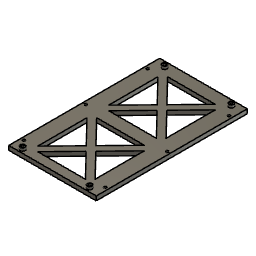
psu_base (Autodesk Fusion 360 design; units mm, degrees)
Autodesk Fusion 360 part; units mm, degrees
sketch "base" plane through (0, 0, 0) normal (0, 1, 0) x (1, 0, 0)
  line L0 (0, 0) -> (125, 0)
  line L1 (0, 0) -> (0, -245)
  line L2 (0, -245) -> (125, -245)
  line L3 (125, -245) -> (125, 0)
  line L4 (125, 0) -> (110, 0) construction
  line L5 (110, 0) -> (110, -15) construction
  line L6 (110, -15) -> (15, -15)
  line L7 (15, -15) -> (15, -230)
  line L8 (15, -230) -> (110, -230)
  line L9 (110, -230) -> (110, -15)
  line L10 (15, -122.5) -> (110, -122.5)
  line L11 (110, -122.5) -> (110, -132.5)
  line L12 (110, -132.5) -> (15, -132.5)
  line L13 (15, -132.5) -> (15, -122.5)
  line L14 (15, -122.5) -> (110, -122.5)
  line L15 (110, -122.5) -> (110, -112.5)
  line L16 (110, -112.5) -> (15, -112.5)
  line L17 (15, -112.5) -> (15, -122.5)
  line L18 (110, -112.5) -> (102, -112.5) construction
  line L19 (110, -112.5) -> (110, -104.5) construction
  line L20 (15, -15) -> (23, -15) construction
  line L21 (15, -15) -> (15, -23) construction
  line L22 (15, -23) -> (102, -112.5)
  line L23 (23, -15) -> (110, -104.5)
  line L24 (110, -15) -> (110, -23) construction
  line L25 (110, -15) -> (102, -15) construction
  line L26 (15, -112.5) -> (23, -112.5) construction
  line L27 (15, -112.5) -> (15, -104.5) construction
  line L28 (110, -23) -> (23, -112.5)
  line L29 (102, -15) -> (15, -104.5)
  line L30 (110, -132.5) -> (102, -132.5) construction
  line L31 (110, -132.5) -> (110, -140.5) construction
  line L32 (15, -132.5) -> (23, -132.5) construction
  line L33 (15, -132.5) -> (15, -140.5) construction
  line L34 (15, -230) -> (15, -222) construction
  line L35 (15, -230) -> (23, -230) construction
  line L36 (110, -230) -> (102, -230) construction
  line L37 (110, -230) -> (110, -222) construction
  line L38 (102, -132.5) -> (15, -222)
  line L39 (23, -230) -> (110, -140.5)
  line L40 (23, -132.5) -> (110, -222)
  line L41 (15, -140.5) -> (102, -230)
  line L42 (0, 0) -> (125, 0)
  line L43 (125, 0) -> (125, 5)
  line L44 (125, 5) -> (0, 5)
  line L45 (0, 5) -> (0, 0)
  dimension "d1" = 125
  dimension "d2" = 245
  dimension "d3" = 125
  dimension "d4" = 15
  dimension "d5" = 15
  dimension "d6" = 95
  dimension "d7" = 215
  dimension "d8" = 10
  dimension "d9" = 10
  dimension "d92" = 8
  dimension "d93" = 8
  dimension "d94" = 8
  dimension "d95" = 8
  dimension "d96" = 8
  dimension "d97" = 8
  dimension "d98" = 8
  dimension "d99" = 8
  dimension "d100" = 8
  dimension "d101" = 8
  dimension "d102" = 8
  dimension "d103" = 8
  dimension "d104" = 8
  dimension "d105" = 8
  dimension "d106" = 8
  dimension "d107" = 8
  dimension "d110" = 5
  constraint coincident L0.start L1.start
  constraint horizontal L0
  constraint perpendicular L0 L1
  constraint perpendicular L1 L2
  constraint perpendicular L3 L4
  constraint perpendicular L4 L5
  constraint horizontal L6
  constraint vertical L7
  constraint horizontal L8
  constraint vertical L9
  constraint horizontal L10
  constraint vertical L11
  constraint horizontal L12
  constraint vertical L13
  constraint midpoint L7 L10.start
  constraint horizontal L14
  constraint vertical L15
  constraint horizontal L16
  constraint vertical L17
  constraint perpendicular L9 L18
  constraint perpendicular L16 L19
  constraint perpendicular L7 L20
  constraint perpendicular L6 L21
  constraint perpendicular L6 L24
  constraint perpendicular L5 L25
  constraint perpendicular L7 L26
  constraint perpendicular L26 L27
  constraint perpendicular L11 L30
  constraint perpendicular L12 L31
  constraint perpendicular L13 L32
  constraint perpendicular L12 L33
  constraint perpendicular L8 L34
  constraint perpendicular L34 L35
  constraint perpendicular L9 L36
  constraint perpendicular L8 L37
  constraint horizontal L42
  constraint vertical L43
  constraint horizontal L44
  constraint vertical L45
  measures "d1" distance of L0.start L0.end
  measures "d2" distance of L0.start L1.end
  measures "d3" distance of L1.end L2.end
  measures "d4" distance of L0.end L4.end
  measures "d5" distance of L4.end L5.end
  measures "d6" distance of L5.end L6.end
  measures "d7" distance of L5.end L8.end
  measures "d8" distance of L10.start L12.end
  measures "d9" distance of L10.start L16.end
  measures "d92" distance of L15.end L18.end
  measures "d93" distance of L15.end L19.end
  measures "d94" distance of L6.end L20.end
  measures "d95" distance of L6.end L21.end
  measures "d96" distance of L5.end L24.end
  measures "d97" distance of L5.end L25.end
  measures "d98" distance of L16.end L26.end
  measures "d99" distance of L16.end L27.end
  measures "d100" distance of L11.end L30.end
  measures "d101" distance of L11.end L31.end
  measures "d102" distance of L12.end L32.end
  measures "d103" distance of L12.end L33.end
  measures "d104" distance of L7.end L34.end
  measures "d105" distance of L7.end L35.end
  measures "d106" distance of L8.end L36.end
  measures "d107" distance of L8.end L37.end
  measures "d110" distance of L0.start L44.end
sketch "bolt" plane through (0, 0, 0) normal (0, 1, 0) x (1, 0, 0)
  line L0 (0, 0) -> (125, 0) construction
  line L1 (0, 0) -> (7.4, 0) construction
  line L2 (7.4, 0) -> (7.4, -4.25) construction
  circle A0 centre (7.4, -4.25) radius 2.125
  line L3 (125, 0) -> (118, 0) construction
  line L4 (118, 0) -> (118, -4.25) construction
  circle A1 centre (118, -4.25) radius 2.125
  circle A2 centre (7.4, -4.25) radius 4
  circle A3 centre (118, -4.25) radius 4
  line L5 (0, -245) -> (7, -245) construction
  line L6 (7, -245) -> (7, -239) construction
  circle A4 centre (7, -239) radius 4
  circle A5 centre (7, -239) radius 2.125
  line L7 (125, -245) -> (118, -245) construction
  line L8 (118, -245) -> (118, -239) construction
  circle A6 centre (118, -239) radius 4
  circle A7 centre (118, -239) radius 2.125
  point P0 (0, -245)
  point P1 (125, -245)
  dimension "d10" = 7.4
  dimension "d11" = 4.25
  dimension "d12" = 4.25
  dimension "d13" = 7
  dimension "d14" = 4.25
  dimension "d15" = 4.25
  dimension "d16" = 8
  dimension "d17" = 8
  dimension "d18" = 7
  dimension "d19" = 6
  dimension "d20" = 8
  dimension "d21" = 4.25
  dimension "d22" = 7
  dimension "d23" = 6
  dimension "d24" = 8
  dimension "d25" = 4.25
  constraint coincident L0.start L1.start
  constraint coincident L0 L1.end
  constraint perpendicular L1 L2
  constraint coincident L2.end A0.centre
  constraint coincident L0.end L3.start
  constraint perpendicular L0 L4
  constraint coincident L4.end A1.centre
  constraint concentric A0 A2
  constraint concentric A1 A3
  constraint coincident P0 L5.start
  constraint perpendicular L5 L6
  constraint coincident L6.end A4.centre
  constraint concentric A4 A5
  constraint coincident P1 L7.start
  constraint perpendicular L7 L8
  constraint coincident L8.end A6.centre
  constraint concentric A6 A7
  measures "d10" distance of L0.start L1.end
  measures "d11" diameter of A0
  measures "d12" distance of L1.end L2.end
  measures "d13" distance of L0.end L3.end
  measures "d14" distance of L3.end L4.end
  measures "d15" diameter of A1
  measures "d16" diameter of A2
  measures "d17" diameter of A3
  measures "d18" distance of P0 L5.end
  measures "d19" distance of L5.end L6.end
  measures "d20" diameter of A4
  measures "d21" diameter of A5
  measures "d22" distance of P1 L7.end
  measures "d23" distance of L7.end L8.end
  measures "d24" diameter of A6
  measures "d25" diameter of A7
extrude "Extrude1" add sketch "base" along normal blind 7 contours L0 L42 L43 L44 L45 | L0 L1 L2 L3 L42 | L7 L9 L10 L14 L15 L16 L17 | L7 L9 L10 L11 L12 L13 L14
extrude "Extrude2" add sketch "bolt" along normal blind 11.5
sketch "nut" plane through (0, 0, 0) normal (0, 1, 0) x (1, 0, 0)
  line L0 (5.0254, -235.3419) -> (2.8447, -238.881)
  line L1 (2.8447, -238.881) -> (4.8193, -242.5391)
  line L2 (4.8193, -242.5391) -> (8.9746, -242.6581)
  line L3 (8.9746, -242.6581) -> (11.1553, -239.119)
  line L4 (11.1553, -239.119) -> (9.1807, -235.4609)
  line L5 (9.1807, -235.4609) -> (5.0254, -235.3419)
  line L6 (115.6997, -235.5374) -> (113.8512, -239.2608)
  line L7 (113.8512, -239.2608) -> (116.1515, -242.7234)
  line L8 (116.1515, -242.7234) -> (120.3003, -242.4626)
  line L9 (120.3003, -242.4626) -> (122.1488, -238.7392)
  line L10 (122.1488, -238.7392) -> (119.8485, -235.2766)
  line L11 (119.8485, -235.2766) -> (115.6997, -235.5374)
  line L12 (3.243, -4.2395) -> (5.3124, -7.8448)
  line L13 (5.3124, -7.8448) -> (9.4694, -7.8553)
  line L14 (9.4694, -7.8553) -> (11.557, -4.2605)
  line L15 (11.557, -4.2605) -> (9.4876, -0.6552)
  line L16 (9.4876, -0.6552) -> (5.3306, -0.6447)
  line L17 (5.3306, -0.6447) -> (3.243, -4.2395)
  line L18 (115.9734, -0.6205) -> (113.8434, -4.1903)
  line L19 (113.8434, -4.1903) -> (115.87, -7.8198)
  line L20 (115.87, -7.8198) -> (120.0266, -7.8795)
  line L21 (120.0266, -7.8795) -> (122.1566, -4.3097)
  line L22 (122.1566, -4.3097) -> (120.13, -0.6802)
  line L23 (120.13, -0.6802) -> (115.9734, -0.6205)
  point P0 (7, -239)
  point P1 (7, -239)
  point P2 (118, -239)
  point P3 (118, -239)
  point P4 (7.4, -4.25)
  point P5 (7.4, -4.25)
  point P6 (118, -4.25)
  point P7 (118, -4.25)
  dimension "d30" = 4.157
  dimension "d31" = 4.157
  dimension "d32" = 4.157
  dimension "d33" = 4.157
  constraint coincident P1 P0
  constraint coincident P3 P2
  constraint coincident P5 P4
  constraint coincident P7 P6
  measures "d30" distance of L0.start P0
  measures "d31" distance of L6.start P3
  measures "d32" distance of L12.start P5
  measures "d33" distance of L18.start P7
extrude "Extrude3" cut sketch "nut" along normal blind 4
extrude "Extrude4" cut sketch "bolt" along normal blind 10 contours A0 | A1 | A5 | A7
sketch "sides" plane through (0, 0, 0) normal (0, 1, 0) x (1, 0, 0)
  line L0 (0, -245) -> (-10, -245)
  line L1 (-10, -245) -> (-10, 0)
  line L2 (-10, 0) -> (0, 0)
  line L3 (0, 0) -> (0, -245)
  line L4 (125, -245) -> (135, -245)
  line L5 (135, -245) -> (135, 0)
  line L6 (135, 0) -> (125, 0)
  line L7 (125, 0) -> (125, -245)
  line L8 (0, 0) -> (-10, 0)
  line L9 (-10, 0) -> (-10, 5)
  line L10 (-10, 5) -> (0, 5)
  line L11 (0, 5) -> (0, 0)
  line L12 (125, 0) -> (135, 0)
  line L13 (135, 0) -> (135, 5)
  line L14 (135, 5) -> (125, 5)
  line L15 (125, 5) -> (125, 0)
  point P0 (0, -245)
  point P1 (125, -245)
  dimension "d66" = 10
  dimension "d67" = 10
  dimension "d111" = 5
  dimension "d112" = 5
  constraint horizontal L0
  constraint vertical L1
  constraint horizontal L2
  constraint vertical L3
  constraint coincident P0 L0.start
  constraint horizontal L4
  constraint vertical L5
  constraint horizontal L6
  constraint vertical L7
  constraint coincident P1 L4.start
  constraint horizontal L8
  constraint vertical L9
  constraint horizontal L10
  constraint vertical L11
  constraint coincident L2.end L3.start
  constraint horizontal L12
  constraint vertical L13
  constraint horizontal L14
  constraint vertical L15
  measures "d66" distance of P0 L0.end
  measures "d67" distance of P1 L4.end
  measures "d111" distance of L2.end L10.end
  measures "d112" distance of L6.end L14.end
extrude "Extrude7" add sketch "sides" along normal blind 7
sketch "crosssupport" plane through (0, 0, 0) normal (0, 1, 0) x (1, 0, 0)
  line L0 (0, 0) -> (0, -245) construction
  line L1 (126.3999, -227.0785) -> (130, -229.157)
  circle A0 centre (130, -225) radius 2.125
  line L2 (135, -245) -> (130, -245) construction
  line L3 (130, -229.157) -> (133.6001, -227.0785)
  line L4 (130, -220.843) -> (126.3999, -222.9215)
  line L5 (130, -245) -> (130, -225) construction
  line L6 (133.6001, -222.9215) -> (130, -220.843)
  line L7 (126.3999, -222.9215) -> (126.3999, -227.0785)
  line L8 (133.6001, -227.0785) -> (133.6001, -222.9215)
  line L9 (-1.3999, -222.9215) -> (-5, -220.843)
  line L10 (-8.6001, -227.0785) -> (-5, -229.157)
  circle A1 centre (-5, -225) radius 2.125
  line L11 (-1.3999, -227.0785) -> (-1.3999, -222.9215)
  line L12 (-10, -245) -> (-5, -245) construction
  line L13 (-5, -245) -> (-5, -225) construction
  line L14 (-5, -229.157) -> (-1.3999, -227.0785)
  line L15 (-8.6001, -222.9215) -> (-8.6001, -227.0785)
  line L16 (-5, -220.843) -> (-8.6001, -222.9215)
  line L17 (-10, -245) -> (-10, 0)
  line L18 (-4.7762, -118.349) -> (-8.4829, -120.2307)
  circle A2 centre (-5, -122.5) radius 2.125
  line L19 (-8.7068, -124.3817) -> (-5.2238, -126.651)
  line L20 (-1.5171, -124.7693) -> (-1.2932, -120.6183)
  line L21 (-10, -122.5) -> (-5, -122.5) construction
  line L22 (-1.2932, -120.6183) -> (-4.7762, -118.349)
  line L23 (-8.4829, -120.2307) -> (-8.7068, -124.3817)
  line L24 (-5.2238, -126.651) -> (-1.5171, -124.7693)
  line L25 (135, -245) -> (135, 0)
  line L26 (133.6578, -120.5249) -> (130.1184, -118.3447)
  line L27 (135, -122.5) -> (130, -122.5) construction
  circle A3 centre (130, -122.5) radius 2.125
  line L28 (133.5394, -124.6802) -> (133.6578, -120.5249)
  line L29 (130.1184, -118.3447) -> (126.4606, -120.3198)
  line L30 (129.8816, -126.6553) -> (133.5394, -124.6802)
  line L31 (126.4606, -120.3198) -> (126.3422, -124.4751)
  line L32 (126.3422, -124.4751) -> (129.8816, -126.6553)
  line L33 (133.6001, -17.9215) -> (130, -15.843)
  line L34 (130, -15.843) -> (126.3999, -17.9215)
  circle A4 centre (130, -20) radius 2.125
  line L35 (130, 0) -> (130, -20) construction
  line L36 (135, 0) -> (130, 0) construction
  line L37 (133.6001, -22.0785) -> (133.6001, -17.9215)
  line L38 (130, -24.157) -> (133.6001, -22.0785)
  line L39 (126.3999, -17.9215) -> (126.3999, -22.0785)
  line L40 (126.3999, -22.0785) -> (130, -24.157)
  circle A5 centre (-5, -20) radius 2.125
  line L41 (-4.974, -15.8431) -> (-8.587, -17.899)
  line L42 (-10, 0) -> (-5, 0) construction
  line L43 (-8.613, -22.056) -> (-5.026, -24.1569)
  line L44 (-1.413, -22.101) -> (-1.387, -17.944)
  line L45 (-5, 0) -> (-5, -20) construction
  line L46 (-1.387, -17.944) -> (-4.974, -15.8431)
  line L47 (-8.587, -17.899) -> (-8.613, -22.056)
  line L48 (-5.026, -24.1569) -> (-1.413, -22.101)
  point P0 (130, -225)
  point P1 (-5, -225)
  point P2 (-10, -122.5)
  point P3 (-5, -122.5)
  point P4 (135, -122.5)
  point P5 (130, -122.5)
  point P6 (130, -20)
  point P7 (130, -20)
  point P8 (-5, -20)
  point P9 (-5, -20)
  dimension "d68" = 5
  dimension "d70" = 4.25
  dimension "d72" = 5
  dimension "d73" = 20
  dimension "d74" = 4.25
  dimension "d75" = 4.157
  dimension "d76" = 5
  dimension "d77" = 4.25
  dimension "d78" = 4.157
  dimension "d79" = 5
  dimension "d80" = 4.25
  dimension "d82" = 5
  dimension "d84" = 4.25
  dimension "d85" = 4.157
  dimension "d86" = 5
  dimension "d87" = 20
  dimension "d88" = 4.25
  dimension "d89" = 4.157
  constraint perpendicular L2 L5
  constraint coincident P0 A0.centre
  constraint perpendicular L12 L13
  constraint coincident P1 A1.centre
  constraint midpoint P2 L17
  constraint coincident P3 A2.centre
  constraint midpoint P4 L25
  constraint coincident P5 L27.end
  constraint perpendicular L35 L36
  constraint coincident P7 P6
  constraint perpendicular L42 L45
  constraint coincident P9 P8
  measures "d68" distance of L2.start L2.end
  measures "d70" diameter of A0
  measures "d72" distance of L12.start L12.end
  measures "d73" distance of L12.end P1
  measures "d74" diameter of A1
  measures "d75" distance of P1 L10.end
  measures "d76" distance of P3 P2
  measures "d77" diameter of A2
  measures "d78" distance of L20.start P3
  measures "d79" distance of P4 P5
  measures "d80" diameter of A3
  measures "d82" distance of L25.end L35.start
  measures "d84" diameter of A4
  measures "d85" distance of L33.end P7
  measures "d86" distance of L17.end L42.end
  measures "d87" distance of L42.end P9
  measures "d88" diameter of A5
  measures "d89" distance of P9 L41.start
extrude "Extrude5" cut sketch "crosssupport" along normal blind 4
extrude "Extrude6" cut sketch "crosssupport" along normal blind 10 contours A0 | A1 | A2 | A3 | A4 | A5
extrude "Extrude8" add sketch "base" along normal blind 7 contours L6 L9 L23 L28 L29 | L6 L7 L22 L23 L29 | L22 L23 L28 L29 | L9 L16 L22 L23 L28 | L7 L16 L22 L28 L29 | L9 L12 L38 L39 L40 | L7 L12 L38 L40 L41 | L8 L9 L39 L40 L41 | L38 L39 L40 L41 | L7 L8 L38 L39 L41
equation "d10 = 4.9 mm + 2.5 mm"
equation "d12 = 1.75 mm + 2.5 mm"
named bodies: "psu_base"
